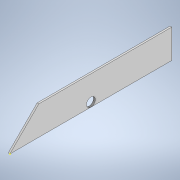
# Autodesk Inventor part: Part7
Saved by Autodesk Inventor 2022 (Build 260153000, 153)
## iProperties
Created: 2021-12-09
Part Number: Part7
Material: Generic
Document SubType Name: Modeling
Designer: keemi
Density: 1 g/cm^3
Appearance: Default
Author: keemi
Autodesk Inventor part; units mm, degrees
ref_plane "YZ Plane" through (0, 0, 0) normal (1, 0, 0) x (0, 1, 0)
ref_plane "XZ Plane" through (0, 0, 0) normal (0, 1, 0) x (-1, 0, 0)
ref_plane "XY Plane" through (0, 0, 0) normal (0, 0, 1) x (1, 0, 0)
sketch "Sketch1" plane through (0, 0, 0) normal (1, 0, 0) x (0, 1, 0)
  line L0 (0, 0) -> (0, -280)
  line L1 (0, -280) -> (50, -280)
  line L2 (50, -280) -> (50, -50)
  line L3 (0, 0) -> (0, 0)
  line L4 (50, -50) -> (0, 0)
  dimension "d0" = 280
  dimension "d1" = 50
  dimension "d2" = 90
  constraints: 10 end point, 3 perpendicular, 1 vertical
  measures "d0" distance of L0.start L0.end
  measures "d1" distance of L0.end L1.end
  measures "d2" angle of L1 L0
extrude "Extrusion1" add sketch "Sketch1" along normal blind 3
sketch "Sketch2" plane through (3, 0, 0) normal (1, 0, 0) x (0, 0, -1)
  line L0 (280, 0) -> (280, 50) projected
  line L1 (280, 50) -> (50, 50) projected
  line L2 (280, 50) -> (140, 50)
  line L3 (140, 50) -> (140, 7.7)
  point P0 (0, 0)
  dimension "d6" = 140
  dimension "d7" = 42.3
  constraints: 4 end point, 1 perpendicular, 1 point on line
  measures "d6" distance of L0.end L2.end
  measures "d7" distance of L2.end L3.end
hole "Hole1" at (3, 7.7, -140) direction (-1, 0, 0) diameter 15.2 end through all
sketch "Sketch3" plane through (3, 0, 0) normal (1, 0, 0) x (0, 0, -1)
  point P0 (0, 0)
body "Solid1"
